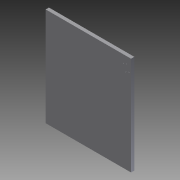
# Autodesk Inventor part: ajustableBase w mounting holes
Saved by Autodesk Inventor 2011 SP1 (Build 150282100, 282)
## iProperties
Created: 2013-01-18
Part Number: ajustableBase w mounting holes
Document SubType Name: Modeling
Designer: wes
Density: 1 g/cm^3
Author: wes
Autodesk Inventor part; units mm, degrees
ref_plane "YZ Plane" through (0, 0, 0) normal (1, 0, 0) x (0, 1, 0)
ref_plane "XZ Plane" through (0, 0, 0) normal (0, 1, 0) x (-1, 0, 0)
ref_plane "XY Plane" through (0, 0, 0) normal (0, 0, 1) x (1, 0, 0)
sketch "Sketch1" plane through (0, 0, 0) normal (0, 0, 1) x (1, 0, 0)
  line L0 (67.8531, 30.0133) -> (728.2531, 30.0133)
  line L1 (728.2531, 30.0133) -> (728.2531, -731.9867)
  line L2 (728.2531, -731.9867) -> (67.8531, -731.9867)
  line L3 (67.8531, -731.9867) -> (67.8531, 30.0133)
  point P0 (0, 0)
  dimension "d0" = 660.4
  dimension "d1" = 762
  constraints: 8 end point, 2 parallel, 1 horizontal, 1 perpendicular
  measures "d0" distance of L0.start L0.end
  measures "d1" distance of L2.end L0.start
extrude "Extrusion1" add sketch "Sketch1" against normal blind 25.4
sketch "Sketch2" plane through (0, 0, 0) normal (0, 0, 1) x (1, 0, 0)
  line L0 (728.2531, 30.0133) -> (728.2531, -731.9867) projected
  line L1 (67.8531, 30.0133) -> (728.2531, 30.0133) projected
  line L2 (670.2463, -29.474) -> (694.1145, -20.7867)
  line L3 (694.1145, -20.7867) -> (711.4891, -68.5231)
  line L4 (711.4891, -68.5231) -> (687.6209, -77.2104)
  line L5 (687.6209, -77.2104) -> (670.2463, -29.474)
  point P0 (0, 0)
  dimension "d29" = 25.4
  dimension "d30" = 50.8
  dimension "d31" = 70
  dimension "d32" = 50.8
  dimension "d33" = 16.764
  constraints: 8 end point, 4 coincident, 2 parallel, 1 perpendicular
  measures "d29" distance between parallel lines of L3 L5
  measures "d30" distance between parallel lines of L4 L2
  measures "d31" angle of L0 L4
  measures "d32" distance from line of L1 L2.end
  measures "d33" distance from line of L0 L3.end
hole "Hole2" at (670.2463, -29.474, 0) at (694.1145, -20.7867, 0) at (711.4891, -68.5231, 0) at (687.6209, -77.2104, 0) direction (0, 0, -1) diameter 6.35 depth 25.4 tip angle 118
body "Solid1"
